Autodesk Inventor part; units mm, degrees
(part 2 of 2)
  spline S265 degree 2 poles (44.5669, -50.5489) (44.0564, -50.5489) (43.0515, -50.9946) (42.5977, -51.4322) knots 0 0 0 1 2 2 2
  line L250 (42.5977, -51.4322) -> (42.5977, -56.7563)
  line L251 (42.5977, -56.7563) -> (41.3336, -56.7563)
  line L252 (41.3336, -56.7563) -> (41.3336, -49.2523)
  line L253 (41.3336, -49.2523) -> (42.5977, -49.2523)
  line L254 (42.5977, -49.2523) -> (42.5977, -50.3706)
  spline S266 degree 2 poles (42.5977, -50.3706) (43.2866, -49.7547) (44.3157, -49.2523) (44.8019, -49.2523) knots 0 0 0 1 2 2 2
  spline S267 degree 2 poles (44.8019, -49.2523) (44.9964, -49.2523) (45.1909, -49.2685) (45.3125, -49.2928) knots 0 0 0 1 2 2 2
  line L255 (45.3125, -49.2928) -> (45.3125, -50.6056)
  line L256 (47.5815, -56.7563) -> (46.3173, -56.7563)
  line L257 (46.3173, -56.7563) -> (46.3173, -49.2523)
  line L258 (46.3173, -49.2523) -> (47.5815, -49.2523)
  line L259 (47.5815, -49.2523) -> (47.5815, -56.7563)
  line L260 (47.6707, -48.0043) -> (46.2363, -48.0043)
  line L261 (46.2363, -48.0043) -> (46.2363, -46.6915)
  line L262 (46.2363, -46.6915) -> (47.6707, -46.6915)
  line L263 (47.6707, -46.6915) -> (47.6707, -48.0043)
  spline S268 degree 2 poles (52.695, -56.9265) (50.896, -56.9265) (48.9186, -54.9087) (48.9186, -53.0448) knots 0 0 0 1 2 2 2
  spline S269 degree 2 poles (48.9186, -53.0448) (48.9186, -51.2134) (50.8392, -49.0416) (52.387, -49.0416) knots 0 0 0 1 2 2 2
  spline S270 degree 2 poles (52.387, -49.0416) (53.084, -49.0416) (54.1618, -49.4468) (54.5588, -49.8763) knots 0 0 0 1 2 2 2
  spline S271 degree 2 poles (54.5588, -49.8763) (54.964, -50.3058) (55.3935, -51.5456) (55.3935, -52.4452) knots 0 0 0 1 2 2 2
  line L264 (55.3935, -52.4452) -> (55.3935, -53.134)
  line L265 (55.3935, -53.134) -> (50.199, -53.134)
  spline S272 degree 2 poles (50.199, -53.134) (50.199, -54.4387) (51.5118, -55.8244) (52.6788, -55.8244) knots 0 0 0 1 2 2 2
  spline S273 degree 2 poles (52.6788, -55.8244) (53.0921, -55.8244) (53.8943, -55.638) (54.2185, -55.4922) knots 0 0 0 1 2 2 2
  spline S274 degree 2 poles (54.2185, -55.4922) (54.5588, -55.3301) (55.0289, -55.0464) (55.1828, -54.9168) knots 0 0 0 1 2 2 2
  line L266 (55.1828, -54.9168) -> (55.2558, -54.9168)
  line L267 (55.2558, -54.9168) -> (55.2558, -56.2944)
  spline S275 degree 2 poles (55.2558, -56.2944) (55.037, -56.3836) (54.3725, -56.6429) (54.1131, -56.7158) knots 0 0 0 1 2 2 2
  spline S276 degree 2 poles (54.1131, -56.7158) (53.7485, -56.8212) (53.1488, -56.9265) (52.695, -56.9265) knots 0 0 0 1 2 2 2
  spline S277 degree 2 poles (54.1618, -52.1696) (54.1455, -51.6591) (53.9349, -50.9135) (53.7323, -50.6623) knots 0 0 0 1 2 2 2
  spline S278 degree 2 poles (53.7323, -50.6623) (53.5135, -50.3787) (52.8246, -50.0789) (52.3141, -50.0789) knots 0 0 0 1 2 2 2
  spline S279 degree 2 poles (52.3141, -50.0789) (51.8117, -50.0789) (51.1066, -50.3787) (50.8149, -50.6704) knots 0 0 0 1 2 2 2
  spline S280 degree 2 poles (50.8149, -50.6704) (50.5313, -50.9703) (50.2396, -51.6915) (50.199, -52.1696) knots 0 0 0 1 2 2 2
  line L268 (50.199, -52.1696) -> (54.1618, -52.1696)
  line L269 (60.6528, -50.6056) -> (60.588, -50.6056)
  spline S281 degree 2 poles (60.588, -50.6056) (60.4421, -50.5651) (60.1261, -50.5489) (59.9073, -50.5489) knots 0 0 0 1 2 2 2
  spline S282 degree 2 poles (59.9073, -50.5489) (59.3968, -50.5489) (58.3919, -50.9946) (57.9381, -51.4322) knots 0 0 0 1 2 2 2
  line L270 (57.9381, -51.4322) -> (57.9381, -56.7563)
  line L271 (57.9381, -56.7563) -> (56.6739, -56.7563)
  line L272 (56.6739, -56.7563) -> (56.6739, -49.2523)
  line L273 (56.6739, -49.2523) -> (57.9381, -49.2523)
  line L274 (57.9381, -49.2523) -> (57.9381, -50.3706)
  spline S283 degree 2 poles (57.9381, -50.3706) (58.6269, -49.7547) (59.6561, -49.2523) (60.1423, -49.2523) knots 0 0 0 1 2 2 2
  spline S284 degree 2 poles (60.1423, -49.2523) (60.3368, -49.2523) (60.5313, -49.2685) (60.6528, -49.2928) knots 0 0 0 1 2 2 2
  line L275 (60.6528, -49.2928) -> (60.6528, -50.6056)
  spline S285 degree 2 poles (63.6593, -56.9346) (62.9057, -56.9346) (61.601, -56.5294) (61.1715, -56.3025) knots 0 0 0 1 2 2 2
  line L276 (61.1715, -56.3025) -> (61.1715, -54.8844)
  line L277 (61.1715, -54.8844) -> (61.2363, -54.8844)
  spline S286 degree 2 poles (61.2363, -54.8844) (61.3984, -55.014) (61.836, -55.322) (62.2007, -55.4922) knots 0 0 0 1 2 2 2
  spline S287 degree 2 poles (62.2007, -55.4922) (62.5167, -55.6461) (63.2947, -55.873) (63.7079, -55.873) knots 0 0 0 1 2 2 2
  spline S288 degree 2 poles (63.7079, -55.873) (64.0078, -55.873) (64.6966, -55.7353) (64.8587, -55.6218) knots 0 0 0 1 2 2 2
  spline S289 degree 2 poles (64.8587, -55.6218) (65.0937, -55.4678) (65.3044, -55.1194) (65.3044, -54.7628) knots 0 0 0 1 2 2 2
  spline S290 degree 2 poles (65.3044, -54.7628) (65.3044, -54.3171) (64.8182, -53.8552) (64.1942, -53.7012) knots 0 0 0 1 2 2 2
  spline S291 degree 2 poles (64.1942, -53.7012) (63.9511, -53.6445) (63.1731, -53.4824) (62.8408, -53.3933) knots 0 0 0 1 2 2 2
  spline S292 degree 2 poles (62.8408, -53.3933) (61.9819, -53.1421) (61.2039, -52.1048) (61.2039, -51.3674) knots 0 0 0 1 2 2 2
  spline S293 degree 2 poles (61.2039, -51.3674) (61.2039, -50.3463) (62.7355, -49.074) (63.9997, -49.074) knots 0 0 0 1 2 2 2
  spline S294 degree 2 poles (63.9997, -49.074) (64.6237, -49.074) (65.8878, -49.3819) (66.3173, -49.617) knots 0 0 0 1 2 2 2
  line L278 (66.3173, -49.617) -> (66.3173, -50.9703)
  line L279 (66.3173, -50.9703) -> (66.2525, -50.9703)
  spline S295 degree 2 poles (66.2525, -50.9703) (65.7663, -50.5813) (64.5831, -50.1356) (63.9754, -50.1356) knots 0 0 0 1 2 2 2
  spline S296 degree 2 poles (63.9754, -50.1356) (63.3514, -50.1356) (62.4924, -50.6623) (62.4924, -51.1891) knots 0 0 0 1 2 2 2
  spline S297 degree 2 poles (62.4924, -51.1891) (62.4924, -51.6672) (63.0029, -52.1291) (63.5702, -52.275) knots 0 0 0 1 2 2 2
  spline S298 degree 2 poles (63.5702, -52.275) (63.8457, -52.3479) (64.5426, -52.4938) (64.9235, -52.5829) knots 0 0 0 1 2 2 2
  spline S299 degree 2 poles (64.9235, -52.5829) (65.7501, -52.7936) (66.5929, -53.758) (66.5929, -54.5926) knots 0 0 0 1 2 2 2
  spline S300 degree 2 poles (66.5929, -54.5926) (66.5929, -55.0789) (66.212, -55.9379) (65.8392, -56.2539) knots 0 0 0 1 2 2 2
  spline S301 degree 2 poles (65.8392, -56.2539) (65.4421, -56.5862) (64.4292, -56.9346) (63.6593, -56.9346) knots 0 0 0 1 2 2 2
  point P0 (43, -56.6301)
  constraints: 2 other
extrude "Extrusion2" cut sketch "Sketch2" against normal blind 1
extrude "Extrusion3" add sketch "Sketch2" along normal blind 0.5
body "Solid1"
